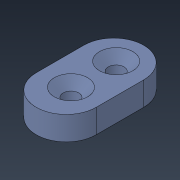
# Autodesk Inventor part: Dribbler Slider
Saved by Autodesk Inventor 2022.1 (Build 261234020, 234B)
## iProperties
Part Number: Dribbler Slider
Material: Gummi, Silikon
Document SubType Name: Modeling
Designer: rYan
Mass: 1.05946 g
Surface Area: 7.33408 cm^2
Volume: 0.847566 cm^3
Density: 1.25 g/cm^3
Appearance: Gummi - Blau
Author: rYan
Autodesk Inventor part; units mm, degrees
ref_plane "YZ Plane" through (0, 0, 0) normal (1, 0, 0) x (0, 1, 0)
ref_plane "XZ Plane" through (0, 0, 0) normal (0, 1, 0) x (-1, 0, 0)
ref_plane "XY Plane" through (0, 0, 0) normal (0, 0, 1) x (1, 0, 0)
sketch "Skizze1" plane through (0, 0, 0) normal (0, 0, 1) x (1, 0, 0)
  line L0 (0, -5) -> (0, 5) construction
  line L1 (6.3, -5) -> (6.3, 5)
  line L2 (-6.3, 5) -> (-6.3, -5)
  arc A0 (-6.3, -5) -> (6.3, -5) centre (0, -5) ccw
  arc A1 (6.3, 5) -> (-6.3, 5) centre (0, 5) ccw
  point P0 (0, 0)
  dimension "d0" = 12.6
  dimension "d1" = 10
  constraints: 8 end point, 4 point on circle, 4 tangent, 2 centre point, 1 midpoint, 1 parallel, 1 vertical
  measures "d0" diameter of A1
  measures "d1" distance of L0.start L0.end
extrude "Extrusion1" add sketch "Skizze1" along normal blind 5
sketch "Skizze2" plane through (0, 0, 5) normal (0, 0, 1) x (1, 0, 0)
  arc A0 (6.3, 5) -> (-6.3, 5) centre (0, 5) ccw projected
  arc A1 (-6.3, -5) -> (6.3, -5) centre (0, -5) ccw projected
  line L0 (0, 5.5) -> (0, -4) construction
  point P0 (0, 0)
  dimension "d11" = 9.5
  dimension "d13" = 1
  constraints: 2 end point, 1 point on line, 1 vertical
  measures "d11" distance of L0.start L0.end
  measures "d13" distance of L0.end A1.centre
hole "Bohrung1" at (0, 5.5, 5) at (0, -4, 5) direction (0, 0, -1) diameter 3.3 end through all countersink diameter 7 countersink angle 90
